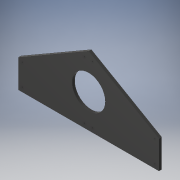
# Autodesk Inventor part: BA10
Saved by Autodesk Inventor 2017 (Build 210142000, 142)
## iProperties
Created: 2018-10-18
Part Number: BA10
Material: ABS Plastic
Document SubType Name: Modeling
Designer: Dell
Density: 1.06 g/cm^3
Appearance: Smooth - Black
Author: Dell
Autodesk Inventor part; units mm, degrees
ref_plane "YZ Plane" through (0, 0, 0) normal (1, 0, 0) x (0, 1, 0)
ref_plane "XZ Plane" through (0, 0, 0) normal (0, 1, 0) x (-1, 0, 0)
ref_plane "XY Plane" through (0, 0, 0) normal (0, 0, 1) x (1, 0, 0)
sketch "Sketch1" plane through (0, 0, 0) normal (0, 0, 1) x (1, 0, 0)
  line L0 (0, 0) -> (505.9426, 0)
  line L1 (505.9426, 0) -> (505.9426, 98.87)
  line L2 (505.9426, 98.87) -> (0, 98.87)
  line L3 (0, 98.87) -> (0, 0)
  line L4 (0, 98.87) -> (252.9713, 244.923)
  line L5 (252.9713, 244.923) -> (505.9426, 98.87)
  point P0 (252.9713, 98.87)
  dimension "d0" = 505.9426
  dimension "d1" = 98.87
  dimension "d2" = 30
  constraints: 12 end point, 2 parallel, 1 horizontal, 1 midpoint, 1 perpendicular, 1 vertical alignment
  measures "d0" distance of L1.end L2.end
  measures "d1" distance of L0.end L1.end
  measures "d2" angle of L2 L5
extrude "Extrusion1" add sketch "Sketch1" along normal blind 10
sketch "Sketch2" plane through (0, 0, 10) normal (0, 0, 1) x (1, 0, 0)
  line L0 (0, 98.87) -> (0, 0) projected
  line L1 (252.9713, 244.923) -> (0, 98.87) projected
  line L2 (505.9426, 98.87) -> (252.9713, 244.923) projected
  line L3 (505.9426, 0) -> (505.9426, 98.87) projected
  line L4 (-10, 0) -> (-10, 104.6435)
  line L5 (-10, 104.6435) -> (252.9713, 256.4701)
  line L6 (252.9713, 256.4701) -> (515.9426, 104.6435)
  line L7 (515.9426, 104.6435) -> (515.9426, 0)
  line L8 (-10, 0) -> (0, 0)
  line L9 (0, 0) -> (505.9426, 0) projected
  line L10 (505.9426, 0) -> (515.9426, 0)
  dimension "d5" = 10
  constraints: 12 end point, 1 collinear, 1 horizontal, 3 other
  measures "d5" distance between parallel lines of L0 L4
extrude "Extrusion2" add sketch "Sketch2" against normal blind 10 contours L0 L8 L4 L5 L6 L7 L10 L3 L2 L1
sketch "Sketch4" plane through (0, 0, 10) normal (0, 0, 1) x (1, 0, 0)
  line L0 (252.9713, 256.4701) -> (-10, 104.6435) construction
  line L1 (-10, 104.6435) -> (-10, 0) construction
  line L2 (-10, 0) -> (515.9426, 0) construction
  line L3 (5, 95.9832) -> (237.9713, 230.4893) construction
  line L4 (237.9713, 230.4893) -> (237.9713, 15) construction
  line L5 (237.9713, 15) -> (5, 15) construction
  line L6 (5, 15) -> (5, 95.9832) construction
  circle A0 centre (5, 15) radius 2.5
  circle A1 centre (5, 95.9832) radius 2.5
  circle A2 centre (237.9713, 230.4893) radius 2.5
  circle A3 centre (237.9713, 15) radius 2.5
  line L7 (515.9426, 0) -> (515.9426, 104.6435) projected
  line L8 (515.9426, 104.6435) -> (252.9713, 256.4701) projected
  point P0 (0, 0)
  dimension "d10" = 15
  dimension "d11" = 5
  dimension "d12" = 5
  dimension "d13" = 5
  dimension "d14" = 5
  constraints: 8 end point, 4 centre point, 4 coincident, 1 other
  measures "d10" distance between parallel lines of L0 L3
  measures "d11" diameter of A0
  measures "d12" diameter of A1
  measures "d13" diameter of A2
  measures "d14" diameter of A3
extrude "Extrusion4" cut sketch "Sketch4" against normal through all
sketch "Sketch6" plane through (0, 0, 10) normal (0, 0, 1) x (1, 0, 0)
  circle A0 centre (5, 95.9832) radius 2.5 projected
  circle A1 centre (5, 15) radius 2.5 projected
  circle A2 centre (237.9713, 15) radius 2.5 projected
  circle A3 centre (237.9713, 230.4893) radius 2.5 projected
  line L0 (252.9713, 256.4701) -> (515.9426, 104.6435) projected
  line L1 (252.9713, 256.4701) -> (252.9713, 0) construction
  line L2 (-10, 0) -> (515.9426, 0) projected
  circle A4 centre (500.9426, 95.9832) radius 2.5
  circle A5 centre (500.9426, 15) radius 2.5
  circle A6 centre (267.9713, 15) radius 2.5
  circle A7 centre (267.9713, 230.4893) radius 2.5
  point P0 (0, 0)
  constraints: 4 centre point, 4 symmetric about line, 2 end point, 1 midpoint, 4 other
extrude "Extrusion6" cut sketch "Sketch6" against normal through all contours A4 | A5 | A6 | A7
sketch "Sketch7" plane through (0, 0, 10) normal (0, 0, 1) x (1, 0, 0)
  circle A0 centre (252.9713, 124.5275) radius 62.5
  point P0 (0, 0)
  point P1 (252.9713, 256.4701)
  dimension "d26" = 125
  dimension "d27" = 131.9426
  constraints: 1 centre point, 1 vertical alignment
  measures "d26" diameter of A0
  measures "d27" distance of point (252.971, 256.47) A0.centre
extrude "Extrusion7" cut sketch "Sketch7" against normal through all
body "Solid1"
